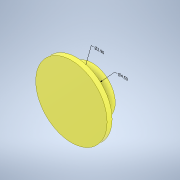
# Autodesk Inventor part: 3inPvcCap
Saved by Autodesk Inventor 2022.2 (Build 262287000, 287)
## iProperties
Created: 2021-11-22
Part Number: 3inPvcCap
Material: PC/ABS Plastic
Document SubType Name: Modeling
Designer: robst
Density: 0.357273 g/cm^3
Appearance: Smooth - Yellow
Author: robst
Autodesk Inventor part; units mm, degrees
ref_plane "YZ Plane" through (0, 0, 0) normal (1, 0, 0) x (0, 1, 0)
ref_plane "XZ Plane" through (0, 0, 0) normal (0, 1, 0) x (-1, 0, 0)
ref_plane "XY Plane" through (0, 0, 0) normal (0, 0, 1) x (1, 0, 0)
sketch "Sketch1" plane through (0, 0, 0) normal (0, 0, 1) x (1, 0, 0)
  circle A0 centre (0, 0) radius 44.45
  circle A1 centre (0, 0) radius 36.83
  circle A2 centre (0, 0) radius 57.15
  circle A3 centre (0, 0) radius 30.48
  dimension "d0" = 88.9
  dimension "d1" = 73.66
  dimension "d4" = 12.7
  dimension "d7" = 6.35
  constraints: 4 centre point, 4 coincident
  measures "d0" diameter of A0
  measures "d1" diameter of A1
  measures "d4" radial gap between concentric circles of A0 A2
  measures "d7" radial gap between concentric circles of A3 A1
extrude "Extrusion2" add sketch "Sketch1" along normal blind 8 contours A0 | A1 | A2 | A3
extrude "Extrusion3" add sketch "Sketch1" against normal blind 25.4 contours A1
sketch "Sketch3" plane through (0, 0, 8) normal (0, 0, 1) x (1, 0, 0)
  ellipse E0 centre (0, 0) end of major axis (57.15, 0) minor radius 60.8178
  circle A0 centre (0, 0) radius 57.15 projected
  circle A1 centre (0, 0) radius 57.15
  point P0 (-57.15, 0)
  point P1 (57.15, 0)
  dimension "d11" = 60.8178
  dimension "d12" = 57.15
  constraints: 2 coincident, 1 centre point, 1 concentric, 2 other
equation "\"d0\" = outsideDiameter"
equation "\"d1\" = insideDiameter"
equation "\"d11\" = 0.5 * elipseMajorDiameter"
equation "\"d12\" = 0.5 * elipseMinorDiameter"
equation "\"insideDiameter\" = 73.66"
equation "\"outsideDiameter\" = 88.9"
equation "\"elipseMajorDiameter\" = 121.63552"
equation "\"elipseMinorDiameter\" = 114.3"
body "Solid2"
